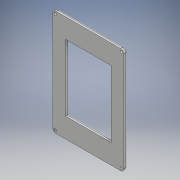
# Autodesk Inventor part: LidTest01
Saved by Autodesk Inventor 2018 (Build 220112000, 112)
## iProperties
Created: 2022-01-12
Part Number: LidTest01
Material: Generic
Document SubType Name: Modeling
Designer: Stewart Alexander
Density: 1 g/cm^3
Appearance: Default
Author: Stewart Alexander
Autodesk Inventor part; units mm, degrees
ref_plane "YZ Plane" through (0, 0, 0) normal (1, 0, 0) x (0, 1, 0)
ref_plane "XZ Plane" through (0, 0, 0) normal (0, 1, 0) x (-1, 0, 0)
ref_plane "XY Plane" through (0, 0, 0) normal (0, 0, 1) x (1, 0, 0)
sketch "Sketch1" plane through (0, 0, 0) normal (0, 1, 0) x (-1, 0, 0)
  line L0 (0, 0) -> (83.3, 0)
  line L1 (83.3, 0) -> (83.3, -124)
  line L2 (83.3, -124) -> (0, -124)
  line L3 (0, -124) -> (0, 0)
  dimension "d0" = 124
  dimension "d1" = 83.3
  constraints: 8 end point, 2 parallel, 1 horizontal, 1 perpendicular
  measures "d0" distance of L0.end L1.end
  measures "d1" distance of L1.end L2.end
extrude "Lid Body" add sketch "Sketch1" along normal blind 4
fillet "4mm Fillet" radius 4 4 edges at (0, 2, -124) (-83.3, 2, -124) (-83.3, 2, 0) (0, 2, 0)
sketch "Sketch2" plane through (0, 4, 0) normal (0, 1, 0) x (1, 0, 0)
  circle A0 centre (-80.3, 3) radius 1.5
  line L0 (-83.3, 124) -> (-83.3, 0) projected
  line L1 (-83.3, 0) -> (0, 0) projected
  line L2 (-83.3, 62) -> (0, 62)
  line L3 (0, 0) -> (0, 124) projected
  line L4 (-41.65, 0) -> (-41.65, 124)
  circle A1 centre (-80.3, 121) radius 1.5
  circle A2 centre (-3, 3) radius 1.5
  circle A3 centre (-3, 121) radius 1.5
  dimension "d5" = 3
  dimension "d6" = 3
  dimension "d7" = 3
  constraints: 4 centre point, 4 end point, 3 midpoint, 3 symmetric about line, 1 vertical, 3 other
  measures "d5" diameter of A0
  measures "d6" distance from line of L0 A0.centre
  measures "d7" distance from line of L1 A0.centre
extrude "Extrusion2" cut sketch "Sketch2" against normal through all contours A0 | A1 | A2 | A3
sketch "Sketch3" plane through (0, 4, 0) normal (0, 1, 0) x (1, 0, 0)
  line L0 (-83.3, 0) -> (0, 0) projected
  line L1 (0, 0) -> (0, 124) projected
  line L2 (0, 124) -> (-83.3, 124) projected
  line L3 (-83.3, 124) -> (-83.3, 0) projected
  line L4 (-78.3, 5) -> (-5, 5)
  line L5 (-5, 5) -> (-5, 119)
  line L6 (-5, 119) -> (-78.3, 119)
  line L7 (-78.3, 119) -> (-78.3, 5)
  line L8 (-68.095, 22.786) -> (-14.795, 22.786)
  line L9 (-14.795, 22.786) -> (-14.795, 100.786)
  line L10 (-14.795, 100.786) -> (-68.095, 100.786)
  line L11 (-68.095, 100.786) -> (-68.095, 22.786)
  dimension "d11" = 5
  dimension "d12" = 53.3
  dimension "d13" = 78
  dimension "d14" = 10.205
  dimension "d15" = 17.786
  constraints: 16 end point, 2 parallel, 1 horizontal, 1 perpendicular, 3 other
  measures "d11" distance between parallel lines of L3 L7
  measures "d12" distance of L9.end L10.end
  measures "d13" distance of L8.end L9.end
  measures "d14" distance between parallel lines of L7 L11
  measures "d15" distance between parallel lines of L4 L8
extrude "Extrusion3" cut sketch "Sketch3" against normal through all contours L11 L10 L9 L8
fillet "2mm Fillet" radius 2 12 edges at (-82.1284, 4, -1.1716) (-41.65, 4, 0) (-1.1716, 4, -1.1716) (0, 4, -62) (-1.1716, 4, -122.8284) (-41.65, 4, -124) (-82.1284, 4, -122.8284) (-83.3, 4, -62) (-68.095, 4, -61.786) (-41.445, 4, -22.786) (-14.795, 4, -61.786) (-41.445, 4, -100.786)
body "Solid1"
